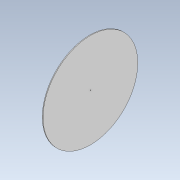
# Autodesk Inventor part: WheelFace
Saved by Autodesk Inventor 2021 (Build 250183000, 183)
## iProperties
Created: 2021-08-28
Part Number: WheelFace
Material: Generic
Document SubType Name: Modeling
Designer: digge
Density: 1 g/cm^3
Appearance: Default
Author: digge
Autodesk Inventor part; units mm, degrees
ref_plane "YZ Plane" through (0, 0, 0) normal (1, 0, 0) x (0, 1, 0)
ref_plane "XZ Plane" through (0, 0, 0) normal (0, 1, 0) x (-1, 0, 0)
ref_plane "XY Plane" through (0, 0, 0) normal (0, 0, 1) x (1, 0, 0)
sketch "Sketch1" plane through (0, 0, 0) normal (1, 0, 0) x (0, 1, 0)
  circle A0 centre (168, 158) radius 175
  circle A1 centre (168, 158) radius 1.5
  point P0 (0, 0)
  dimension "d0" = 3
  dimension "d1" = 350
  constraints: 2 centre point, 1 coincident
  measures "d0" diameter of A1
  measures "d1" diameter of A0
extrude "Extrusion1" add sketch "Sketch1" along normal blind 3
equation "\"d0\" = ScrewDiameter"
equation "\"d1\" = WheelDiameter"
equation "\"d2\" = Width"
equation "\"WheelDiameter\" = 350"
equation "\"ScrewDiameter\" = 3"
equation "\"Width\" = 3"
body "Solid1"
